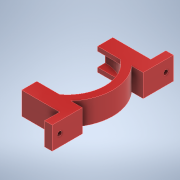
# Autodesk Inventor part: LensSupport
Saved by Autodesk Inventor 2022.2 (Build 262287010, 287A)
## iProperties
Created: 2022-05-11
Part Number: LensSupport
Material: Plástico ABS
Document SubType Name: Modeling
Designer: mabel
Density: 1.06 g/cm^3
Appearance: Rojo
Author: mabel
Autodesk Inventor part; units mm, degrees
ref_plane "YZ Plane" through (0, 0, 0) normal (1, 0, 0) x (0, 1, 0)
ref_plane "XZ Plane" through (0, 0, 0) normal (0, 1, 0) x (-1, 0, 0)
ref_plane "XY Plane" through (0, 0, 0) normal (0, 0, 1) x (1, 0, 0)
sketch "Boceto1" plane through (0, 0, 0) normal (0, 1, 0) x (-1, 0, 0)
  arc A0 (0, 25.125) -> (0, -25.125) centre (0, 0) ccw
  arc A1 (0, 30.125) -> (0, -30.125) centre (0, 0) ccw
  line L0 (0, 30.125) -> (-30.125, 30.125)
  line L1 (-30.125, 30.125) -> (-30.125, 20.125)
  line L2 (-30.125, 20.125) -> (-22.4165, 20.125)
  line L3 (6.35, 0) -> (-9.525, 0)
  line L4 (0, -30.125) -> (-30.125, -30.125)
  line L5 (-30.125, -30.125) -> (-30.125, -20.125)
  line L6 (-30.125, -20.125) -> (-22.4165, -20.125)
  line L7 (0, 30.125) -> (0, 25.125)
  line L8 (0, -25.125) -> (0, -30.125)
  dimension "d0" = 50.25
  dimension "d1" = 5
  dimension "d2" = 10
  constraints: 18 end point, 5 point on circle, 4 symmetric about line, 2 centre point, 2 horizontal, 2 perpendicular, 2 vertical, 1 coincident, 1 tangent
  measures "d0" diameter of A0
  measures "d1" radial gap between concentric circles of A0 A1
  measures "d2" distance of L0.end L1.end
extrude "Extrusión1" add sketch "Boceto1" along normal blind 15
sketch "Boceto2" plane through (0, 15, 0) normal (0, 1, 0) x (1, 0, 0)
  arc A0 (0, -25.125) -> (0, 25.125) centre (0, 0) ccw projected
  line L0 (0, 25.125) -> (0, 20.125)
  line L1 (0, 20.125) -> (15.0416, 20.125)
  dimension "d5" = 5
  constraints: 4 end point, 1 perpendicular, 1 point on circle, 1 vertical
  measures "d5" distance of L0.start L0.end
extrude "Extrusión2" add sketch "Boceto2" against normal blind 2.95
mirror "Simetría1" about plane through (0, 0, 0) normal (0, 0, 1) of "Extrusión2"
sketch "Boceto3" plane through (0, 0, 0) normal (0, -1, 0) x (1, 0, 0)
  arc A0 (0, -25.125) -> (15.0416, -20.125) centre (0, 0) ccw projected
  line L0 (0, -20.125) -> (0, -25.125) projected
  line L1 (0, -25.125) -> (0, -20.125)
  line L2 (0, -20.125) -> (15.0416, -20.125)
  constraints: 4 end point, 1 collinear, 1 perpendicular
extrude "Extrusión3" add sketch "Boceto3" against normal blind 2.95
mirror "Simetría2" about plane through (0, 0, 0) normal (0, 0, 1) of "Extrusión3"
sketch "Boceto4" plane through (0, 0, 30.125) normal (0, 0, 1) x (1, 0, 0)
  line L0 (30.125, 0) -> (30.125, 15) projected
  line L1 (30.125, 15) -> (25.125, 15)
  line L2 (25.125, 15) -> (25.125, 0)
  line L3 (25.125, 0) -> (30.125, 0)
  line L4 (30.125, 0) -> (30.125, 15)
  point P0 (0, 0)
  dimension "d10" = 5
  constraints: 8 end point, 2 parallel, 1 horizontal, 1 perpendicular, 1 point on line
  measures "d10" distance of L3.end L2.end
extrude "Extrusión4" add sketch "Boceto4" along normal blind 10
sketch "Boceto5" plane through (25.125, 0, 30.125) normal (-1, 0, 0) x (0, 0, 1)
  line L0 (-10, 15) -> (10, 15) projected
  line L1 (-10, 0) -> (0, 0) projected
  line L2 (10, 15) -> (0, 15)
  line L3 (0, 15) -> (0, 0)
  line L4 (0, 0) -> (10, 0)
  line L5 (10, 0) -> (10, 15)
  circle A0 centre (5, 7.5) radius 1.5
  point P0 (-30.125, 0)
  dimension "d13" = 3
  constraints: 8 end point, 2 parallel, 1 centre point, 1 horizontal, 1 perpendicular
  measures "d13" diameter of A0
extrude "Extrusión5" cut sketch "Boceto5" against normal blind 10 contours A0
mirror "Simetría3" about plane through (0, 0, 0) normal (0, 0, 1) of "Extrusión4", "Extrusión5"
